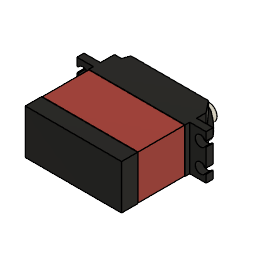
40KgServoMotor_v2 (Autodesk Fusion 360 design; units mm, degrees)
Autodesk Fusion 360 part; units mm, degrees
sketch "Sketch1" plane through (0, 0, 0) normal (0, 0, 1) x (1, 0, 0)
  line L0 (-53, 17) -> (-12, 17)
  line L1 (-12, 17) -> (-12, -24)
  line L2 (-12, -24) -> (-53, -24)
  line L3 (-53, -24) -> (-53, 17)
  line L4 (-53, 5) -> (-60, 5)
  line L5 (-60, 5) -> (-60, 8)
  line L6 (-60, 8) -> (-53, 8)
  line L7 (-32.5, 17) -> (-32.5, 13) construction
  line L8 (-5, 8) -> (-12, 8)
  line L9 (-5, 5) -> (-5, 8)
  line L10 (-12, 5) -> (-5, 5)
  line L11 (-53, 14) -> (-50, 14)
  line L12 (-50, 14) -> (-49, 17)
  line L13 (-12, 12) -> (-16, 17)
  dimension "d2" = 41
  dimension "d3" = 41
  dimension "d4" = 3
  dimension "d5" = 29
  dimension "d6" = 55
  constraint horizontal L0
  constraint vertical L1
  constraint horizontal L2
  constraint vertical L3
  constraint coincident L3 L4.start
  constraint perpendicular L3 L4
  constraint perpendicular L4 L5
  constraint coincident L3 L6.end
  constraint perpendicular L3 L6
  constraint midpoint L0 L7.start
  constraint perpendicular L0 L7
  constraint symmetric L4.start L7 L10.start
  constraint symmetric L4.end L7 L9.start
  constraint symmetric L5.end L7 L8.start
  constraint symmetric L6.end L7 L8.end
  constraint coincident L3 L11.start
  constraint perpendicular L3 L11
  constraint coincident L0 L12.end
  constraint coincident L1 L13.start
  constraint coincident L0 L13.end
  measures "d2" distance of L1.end L2.end
  measures "d3" distance of L0.start L2.end
  measures "d4" distance of L4.end L5.end
  measures "d5" distance of L2 L4
  measures "d6" distance of L5 L9
extrude "Extrude1" add sketch "Sketch1" along normal blind 19 contours L0 L1 L2 L3 L11 L12 L13 | L3 L4 L5 L6 | L1 L8 L9 L10
ref_plane "WorkPlane1" through (-32.5, 17, 9.5) normal (0, 1, 0) x (-1, 0, 0)
sketch "Sketch3" plane through (0, 17, 0) normal (0, 1, 0) x (-1, 0, 0)
  line L0 (16, 0) -> (49, 0)
  line L1 (49, 0) -> (49, 19)
  line L2 (49, 19) -> (16, 19)
  line L3 (16, 19) -> (16, 0)
  circle A0 centre (21.2968, 9.5) radius 3.5
  line L4 (16, 9.5) -> (49, 9.5) construction
  circle A1 centre (21.2968, 9.5) radius 7.55
  circle A2 centre (7.3647, 4.4269) radius 2.25
  line L5 (5.4122, 3.3087) -> (5, 3.3087)
  line L6 (7.3647, 4.4269) -> (5, 4.4269) construction
  line L7 (5, 4.4269) -> (5, 3.3087)
  line L8 (5.4122, 5.5451) -> (5, 5.5451)
  line L9 (5, 4.4269) -> (5, 5.5451)
  circle A3 centre (7.3647, 14.4269) radius 2.25
  line L10 (5.4122, 15.5451) -> (5, 15.5451)
  line L11 (5, 14.4269) -> (5, 15.5451)
  line L12 (7.3647, 14.4269) -> (5, 14.4269) construction
  line L13 (5.4122, 13.3087) -> (5, 13.3087)
  line L14 (5, 14.4269) -> (5, 13.3087)
  line L15 (5, 4.4269) -> (5, 5.5451)
  line L16 (5, 4.4269) -> (5, 3.3087)
  line L17 (5, 14.4269) -> (5, 13.3087)
  line L18 (5.4122, 5.5451) -> (5, 5.5451)
  circle A4 centre (7.3647, 14.4269) radius 2.25
  line L19 (5.4122, 3.3087) -> (5, 3.3087)
  line L20 (7.3647, 14.4269) -> (5, 14.4269) construction
  line L21 (5.4122, 13.3087) -> (5, 13.3087)
  circle A5 centre (7.3647, 4.4269) radius 2.25
  line L22 (5, 14.4269) -> (5, 15.5451)
  line L23 (5.4122, 15.5451) -> (5, 15.5451)
  line L24 (7.3647, 4.4269) -> (5, 4.4269) construction
  line L25 (57.5, 4.4269) -> (60.0092, 4.4269) construction
  line L26 (59.4525, 5.5451) -> (60.0093, 5.5451)
  line L27 (57.5, 14.4269) -> (59.8647, 14.4269) construction
  circle A6 centre (57.5, 4.4269) radius 2.25
  line L28 (59.8647, 14.4269) -> (59.8647, 13.3087)
  line L29 (59.4525, 15.5451) -> (60.0263, 15.5462)
  line L30 (59.4525, 13.3087) -> (60.0263, 13.3076)
  line L31 (60.0284, 14.4269) -> (60.0263, 15.5462)
  line L32 (59.4525, 15.5451) -> (59.8647, 15.5451)
  circle A7 centre (57.5, 14.4269) radius 2.25
  circle A8 centre (57.5, 4.4269) radius 2.25
  line L33 (59.4525, 3.3087) -> (60.0093, 3.3087)
  line L34 (59.8647, 14.4269) -> (59.8647, 15.5451)
  line L35 (60.0284, 14.4269) -> (60.0263, 13.3076)
  line L36 (59.4525, 5.5451) -> (60.0092, 5.5451)
  line L37 (60.0092, 4.4269) -> (60.0092, 3.3086)
  line L38 (57.5, 14.4269) -> (60.0284, 14.4269) construction
  line L39 (59.4525, 13.3087) -> (59.8647, 13.3087)
  line L40 (59.4525, 3.3087) -> (60.0092, 3.3086)
  line L41 (60.0092, 4.4269) -> (60.0093, 5.5451)
  line L42 (57.5, 4.4269) -> (60.0092, 4.4269) construction
  circle A9 centre (57.5, 14.4269) radius 2.25
  line L43 (60.0092, 4.4269) -> (60.0092, 5.5451)
  line L44 (60.0092, 4.4269) -> (60.0093, 3.3087)
  dimension "d10" = 7
  dimension "d11" = 4.5
  dimension "d13" = 4.5
  dimension "d14" = 4.5
  dimension "d15" = 4.5
  dimension "d16" = 4.5
  dimension "d17" = 4.5
  dimension "d18" = 4.5
  dimension "d19" = 4.5
  constraint midpoint L3 L4.start
  constraint midpoint L1 L4.end
  constraint coincident A0.centre L4
  constraint concentric A0 A1
  constraint coincident A2 L5.start
  constraint horizontal L5
  constraint coincident A2.centre L6.start
  constraint horizontal L6
  constraint perpendicular L5 L7
  constraint symmetric L5.start L6 L8.start
  constraint symmetric L5.end L6 L8.end
  constraint symmetric L7.start L6 L9.start
  constraint coincident L13.start A3
  constraint horizontal L13
  constraint coincident A3.centre L12.start
  constraint horizontal L12
  constraint perpendicular L13 L14
  constraint symmetric L10.start L13.start L12
  constraint symmetric L10.end L13.end L12
  constraint symmetric L11.start L14.start L12
  constraint coincident L5.start A5
  constraint horizontal L19
  constraint horizontal L24
  constraint perpendicular L16 L19
  constraint symmetric L8.start L5.start L24
  constraint symmetric L8.end L5.end L24
  constraint symmetric L6.end L7.start L24
  constraint coincident L13.start A4
  constraint horizontal L21
  constraint horizontal L20
  constraint perpendicular L17 L21
  constraint symmetric L13.start L10.start L20
  constraint symmetric L10.end L13.end L20
  constraint symmetric L11.start L12.end L20
  constraint coincident L29.start A9
  constraint coincident L27.start A7.centre
  constraint perpendicular L32 L34
  constraint symmetric L30.start L29.start L27
  constraint symmetric L28.end L32.end L27
  constraint symmetric L28.start L34.start L27
  constraint coincident L26.start A6
  constraint coincident L25.start A6.centre
  constraint perpendicular L36 L43
  constraint symmetric L26.start L33.start L25
  constraint symmetric L37.end L36.end L25
  constraint coincident L29.start A7
  constraint perpendicular L29 L31
  constraint symmetric L30.start L29.start L38
  constraint symmetric L30.end L29.end L38
  constraint coincident L26.start A8
  constraint perpendicular L26 L41
  constraint symmetric L33.start L26.start L42
  constraint symmetric L33.end L26.end L42
  constraint symmetric L25.end L37.start L42
  measures "d10" diameter of A0
  measures "d11" diameter of A2
  measures "d13" diameter of A3
  measures "d14" diameter of A5
  measures "d15" diameter of A4
  measures "d16" diameter of A9
  measures "d17" diameter of A6
  measures "d18" diameter of A7
  measures "d19" diameter of A8
extrude "Extrude2" cut sketch "Sketch3" against normal blind 12 contours A2 A5 | A2 L5 L7 L8 L9 L15 L16 L18 L19 A5 | A3 A4 | A3 L10 L11 L13 L14 L17 A4 L21 L22 L23 | L26 A6 A8 L33 L36 L37 L40 L41 L43 L44 | A6 A8 | L28 L29 L30 L31 L34 L35 | L28 L29 L30 L32 A7 L34 L39 A9 | A7 A9
extrude "Extrude3" add sketch "Sketch3" along normal blind 1 contours L3 A1 | A0 picked at (16.5989, 9.5)
extrude "Extrude4" add sketch "Sketch3" along normal blind 5.5 contours A0
extrude "Extrude5" add sketch "Sketch3" against normal blind 4 contours L3 A1 picked at (14.6309, 10.3442)
chamfer "Chamfer1" distance 2.253 distance2 1 1 edges at (-16, 17, 9.5) measured on face at (-14.6309, 17, 10.3442) tangent chain off
sketch "Sketch4" plane through (0, 8, 0) normal (0, 1, 0) x (-1, 0, 0)
  line L0 (60, 13.3077) -> (59.4525, 13.3087)
  arc A0 (59.4525, 15.5451) -> (59.4525, 13.3087) centre (57.5, 14.4269) ccw
  line L1 (59.4525, 15.5451) -> (60, 15.5461)
  line L2 (60, 15.5461) -> (60, 19)
  line L3 (60, 19) -> (53, 19)
  line L4 (53, 19) -> (53, 0)
  line L5 (53, 0) -> (60, 0)
  line L6 (60, 0) -> (60, 3.3087)
  line L7 (60, 3.3087) -> (59.4525, 3.3087)
  arc A1 (59.4525, 5.5451) -> (59.4525, 3.3087) centre (57.5, 4.4269) ccw
  line L8 (59.4525, 5.5451) -> (60, 5.5451)
  line L9 (60, 5.5451) -> (60, 13.3077)
  line L10 (53, 9.5) -> (59, 9.5) construction
  line L11 (59, 8.5) -> (59, 10.5)
  line L12 (59, 8.5) -> (53, 8.5)
  line L13 (59, 10.5) -> (53, 10.5)
  dimension "d42" = 2
  constraint midpoint L4 L10.start
  constraint perpendicular L4 L10
  constraint midpoint L10.end L11
  constraint perpendicular L10 L11
  constraint perpendicular L11 L12
  constraint coincident L4 L13.end
  constraint perpendicular L4 L13
  measures "d42" distance of L11.start L11.end
extrude "Extrude6" add sketch "Sketch4" along normal blind 2 contours L4 L11 L12 L13
chamfer "Chamfer2" distance 6 distance2 2 1 edges at (-59, 10, 9.5) measured on face at (-55, 10, 9.8333) tangent chain off
sketch "Sketch5" plane through (0, 8, 0) normal (0, 1, 0) x (-1, 0, 0)
  line L0 (5.4122, 13.3087) -> (5, 13.3087)
  line L1 (5, 13.3087) -> (5, 5.5451)
  line L2 (5, 5.5451) -> (5.4122, 5.5451)
  arc A0 (5.4122, 3.3087) -> (5.4122, 5.5451) centre (7.3647, 4.4269) ccw
  line L3 (5.4122, 3.3087) -> (5, 3.3087)
  line L4 (5, 3.3087) -> (5, 0)
  line L5 (5, 0) -> (12, 0)
  line L6 (12, 0) -> (12, 19)
  line L7 (12, 19) -> (5, 19)
  line L8 (5, 19) -> (5, 15.5451)
  line L9 (5, 15.5451) -> (5.4122, 15.5451)
  arc A1 (5.4122, 13.3087) -> (5.4122, 15.5451) centre (7.3647, 14.4269) ccw
  line L10 (12, 9.5) -> (6, 9.5) construction
  line L11 (6, 8.5) -> (6, 10.5)
  line L12 (6, 8.5) -> (12, 8.5)
  line L13 (6, 10.5) -> (12, 10.5)
  constraint midpoint L6 L10.start
  constraint perpendicular L6 L10
  constraint midpoint L10.end L11
  constraint perpendicular L10 L11
  constraint coincident L6 L12.end
  constraint perpendicular L6 L12
  constraint coincident L6 L13.end
  constraint perpendicular L6 L13
extrude "Extrude7" add sketch "Sketch5" along normal blind 2 contours L6 L11 L12 L13
chamfer "Chamfer3" distance 6 distance2 2 1 edges at (-6, 10, 9.5) measured on face at (-8, 10, 9.8333) tangent chain off
sketch "Sketch6" plane through (0, 0, 19) normal (0, 0, 1) x (-1, 0, 0)
  line L0 (12, -5) -> (5, -5)
  line L1 (5, -5) -> (5, -8)
  line L2 (5, -8) -> (12, -8)
  line L3 (12, -8) -> (12, -12)
  line L4 (12, -12) -> (16, -17)
  line L5 (16, -17) -> (49, -17)
  line L6 (49, -17) -> (50, -14)
  line L7 (50, -14) -> (53, -14)
  line L8 (53, -14) -> (53, -8)
  line L9 (53, -8) -> (60, -8)
  line L10 (60, -8) -> (60, -5)
  line L11 (60, -5) -> (53, -5)
  line L12 (53, -5) -> (53, 24)
  line L13 (53, 24) -> (12, 24)
  line L14 (12, 24) -> (12, -5)
  line L15 (53, 17) -> (12, 17)
  line L16 (12, -3) -> (53, -3)
  line L17 (53, -3) -> (52.9, -3)
  line L18 (53, 17) -> (52.9, 17)
  line L19 (52.9, 17) -> (52.9, -3)
  line L20 (12, 17) -> (12.1, 17)
  line L21 (12, -3) -> (12.1, -3)
  line L22 (12.1, -3) -> (12.1, 17)
  dimension "d43" = 0.1
  dimension "d44" = 0.1
  dimension "d45" = 0.1
  dimension "d46" = 0.1
  constraint coincident L12 L15.start
  constraint coincident L14 L15.end
  constraint perpendicular L14 L15
  constraint coincident L14 L16.start
  constraint coincident L12 L16.end
  constraint perpendicular L12 L16
  constraint horizontal L17
  constraint horizontal L18
  constraint horizontal L20
  constraint horizontal L21
  measures "d43" distance of L16.end L17.end
  measures "d44" distance of L15.start L18.end
  measures "d45" distance of L15.end L20.end
  measures "d46" distance of L16.start L21.end
extrude "Extrude8" cut sketch "Sketch6" against normal blind 0.1 contours L15 L16 L19 L22
extrude "Extrude9" cut sketch "Sketch6" against normal blind 19 contours L14 L15 L16 L20 L21 L22 | L12 L15 L16 L17 L18 L19
sketch "Sketch7" plane through (0, 0, 0) normal (0, 0, -1) x (1, 0, 0)
  line L0 (-12, -3) -> (-12.1, -3)
  line L1 (-12.1, -3) -> (-12.1, 17)
  line L2 (-12.1, 17) -> (-12, 17)
  line L3 (-12, 17) -> (-12, 24)
  line L4 (-12, 24) -> (-53, 24)
  line L5 (-53, 24) -> (-53, 17)
  line L6 (-53, 17) -> (-52.9, 17)
  line L7 (-52.9, 17) -> (-52.9, -3)
  line L8 (-52.9, -3) -> (-53, -3)
  line L9 (-53, -3) -> (-53, -5)
  line L10 (-53, -5) -> (-60, -5)
  line L11 (-60, -5) -> (-60, -8)
  line L12 (-60, -8) -> (-53, -8)
  line L13 (-53, -8) -> (-53, -14)
  line L14 (-53, -14) -> (-50, -14)
  line L15 (-50, -14) -> (-49, -17)
  line L16 (-49, -17) -> (-16, -17)
  line L17 (-16, -17) -> (-12, -12)
  line L18 (-12, -12) -> (-12, -8)
  line L19 (-12, -8) -> (-5, -8)
  line L20 (-5, -8) -> (-5, -5)
  line L21 (-5, -5) -> (-12, -5)
  line L22 (-12, -5) -> (-12, -3)
  line L23 (-52.9, 17) -> (-12.1, 17)
  line L24 (-12.1, -3) -> (-52.9, -3)
  constraint coincident L6.end L7.start
  constraint coincident L1.end L2.start
  constraint coincident L0.end L1.start
  constraint coincident L7.end L8.start
extrude "Extrude10" cut sketch "Sketch7" against normal blind 0.1 contours L1 L7 L23 L24
equation "d4 = 32 mm - 29 mm"
